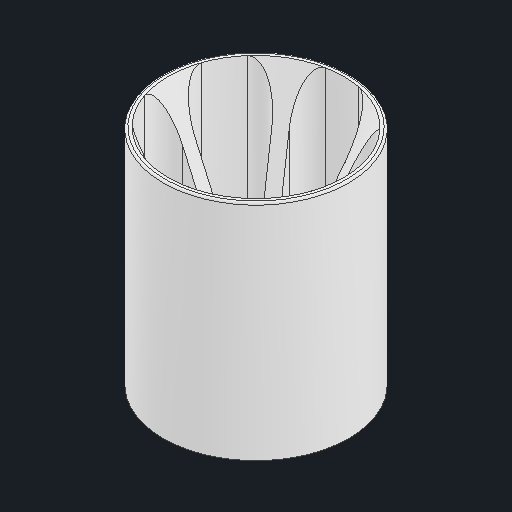
# Autodesk Inventor part: felga
Saved by Autodesk Inventor 2023 (Build 270158000, 158)
## iProperties
Created: 2024-06-08
Part Number: felga
Material: ABS Plastic
Document SubType Name: Modeling
Designer: szymo
Density: 1.06 g/cm^3
Appearance: Smooth - White
Mass: 25.2568 g
Surface Area: 203.005 cm^2
Volume: 23.8272 cm^3
Author: szymo
Autodesk Inventor part; units mm, degrees
ref_plane "YZ Plane" through (0, 0, 0) normal (1, 0, 0) x (0, 1, 0)
ref_plane "XZ Plane" through (0, 0, 0) normal (0, 1, 0) x (-1, 0, 0)
ref_plane "XY Plane" through (0, 0, 0) normal (0, 0, 1) x (1, 0, 0)
sketch "Sketch1" plane through (0, 0, 0) normal (0, 1, 0) x (-1, 0, 0)
  circle A0 centre (0, 0) radius 25
  circle A1 centre (0, 0) radius 22
  circle A2 centre (0, 0) radius 20.8
  dimension "d0" = 50
  dimension "d1" = 3
  dimension "d2" = 1.2
  constraints: 3 centre point, 3 coincident
  measures "d0" diameter of A0
  measures "d1" radial gap between concentric circles of A0 A1
  measures "d2" radial gap between concentric circles of A1 A2
extrude "Extrusion1" add sketch "Sketch1" along normal blind 53 contours A1
sketch "Sketch2" plane through (0, 0, 0) normal (0, 1, 0) x (-1, 0, 0)
  circle A0 centre (0, 0) radius 22 projected
  circle A1 centre (0, 0) radius 20.8 projected
  circle A2 centre (0, 0) radius 5
  line L0 (0, 0) -> (20.8, 0) construction
  circle A3 centre (0, 0) radius 20.8 projected
  line L1 (4.7697, 1.5) -> (20.7458, 1.5)
  line L2 (20.7458, -1.5) -> (4.7697, -1.5)
  line L3 (1.0858, 4.8807) -> (9.0739, 18.7164)
  line L4 (0, 0) -> (10.4, 18.0133) construction
  line L5 (11.672, 17.2164) -> (3.6839, 3.3807)
  line L6 (-3.6839, 3.3807) -> (-11.672, 17.2164)
  line L7 (0, 0) -> (-10.4, 18.0133) construction
  line L8 (-9.0739, 18.7164) -> (-1.0858, 4.8807)
  line L9 (-4.7697, -1.5) -> (-20.7458, -1.5)
  line L10 (0, 0) -> (-20.8, 0) construction
  line L11 (-20.7458, 1.5) -> (-4.7697, 1.5)
  line L12 (-1.0858, -4.8807) -> (-9.0739, -18.7164)
  line L13 (0, 0) -> (-10.4, -18.0133) construction
  line L14 (-11.672, -17.2164) -> (-3.6839, -3.3807)
  line L15 (3.6839, -3.3807) -> (11.672, -17.2164)
  line L16 (0, 0) -> (10.4, -18.0133) construction
  line L17 (9.0739, -18.7164) -> (1.0858, -4.8807)
  point P0 (3.6839, 3.3807)
  point P1 (11.672, 17.2164)
  point P2 (9.0739, 18.7164)
  point P3 (1.0858, 4.8807)
  point P4 (-1.0858, 4.8807)
  point P5 (-9.0739, 18.7164)
  point P6 (-11.672, 17.2164)
  point P7 (-3.6839, 3.3807)
  point P8 (-4.7697, 1.5)
  point P9 (-20.7458, 1.5)
  point P10 (-4.7697, -1.5)
  point P11 (-3.6839, -3.3807)
  point P12 (-9.0739, -18.7164)
  point P13 (-1.0858, -4.8807)
  point P14 (1.0858, -4.8807)
  point P15 (9.0739, -18.7164)
  point P16 (3.6839, -3.3807)
  dimension "d5" = 10
  dimension "d6" = 1.5
  dimension "d7" = 1.5
  dimension "d10" = 360
  constraints: 36 end point, 5 point on circle, 2 parallel, 1 centre point, 1 coincident, 1 horizontal, 55 other
  measures "d5" diameter of A2
  measures "d6" distance between parallel lines of L1 L0
  measures "d7" distance between parallel lines of L0 L2
extrude "Extrusion2" add sketch "Sketch2" along normal blind 17 contours A1 L2 A2 L1 | L5 A2 L3 A1 | A2 | A1 L17 A2 L15 | L8 A2 L6 A1 | A1 L14 A2 L12 | L11 A2 L9 A1
chamfer "Chamfer1" distance 36 distance2 15.8 7 edges at (10.4, 17, 18.0133) (20.8, 17, 0) (10.4, 17, -18.0133) (-10.4, 17, -18.0133) (-20.7865, 17, 0.7505) (-20.7865, 17, -0.7505) (-10.4, 17, 18.0133) measured on face at (10.4, 17.5, 18.0133) measured on face at (-10.4, 17.5, -18.0133) measured on face at (-20.7865, 17.5, -0.7505) measured on face at (-20.7865, 17.5, 0.7505) measured on face at (20.8, 17.5, 0) measured on face at (-10.4, 17.5, 18.0133) measured on face at (10.4, 17.5, -18.0133)
sketch "Sketch3" plane through (0, 0, 0) normal (0, -1, 0) x (1, 0, 0)
  circle A0 centre (0, 0) radius 3
  line L0 (-2.0396, 2.2) -> (2.0396, 2.2)
  line L1 (2.0396, -2.2) -> (-2.0396, -2.2)
  dimension "d19" = 6
  dimension "d20" = 4.4
  dimension "d21" = 2.2
  dimension "d22" = 2.2
  constraints: 4 end point, 4 point on circle, 1 centre point, 1 coincident, 1 horizontal, 1 parallel
  measures "d19" diameter of A0
  measures "d20" distance between parallel lines of L0 L1
  measures "d21" distance from line of L0 point (0, 0)
  measures "d22" distance from line of L1 point (0, 0)
extrude "Extrusion3" cut sketch "Sketch3" against normal blind 12 contours A0 L1 L0
sketch "Sketch6" plane through (0, 0, 0) normal (0, -1, 0) x (1, 0, 0)
  circle A0 centre (0, 0) radius 22 projected
  circle A1 centre (0, -10) radius 3.5
  arc A2 (-9.0739, -18.7164) -> (9.0739, -18.7164) centre (0, 0) ccw projected
  arc A3 (-9.0739, -18.7164) -> (9.0739, -18.7164) centre (0, 0) ccw projected
  circle A4 centre (0, -14.8667) radius 5.9333
  circle A5 centre (12.8749, -7.4333) radius 5.9333
  circle A6 centre (8.6603, -5) radius 3.5
  circle A7 centre (12.8749, 7.4333) radius 5.9333
  circle A8 centre (8.6603, 5) radius 3.5
  circle A9 centre (0, 14.8667) radius 5.9333
  circle A10 centre (0, 10) radius 3.5
  circle A11 centre (-12.8749, 7.4333) radius 5.9333
  circle A12 centre (-8.6603, 5) radius 3.5
  circle A13 centre (-12.8749, -7.4333) radius 5.9333
  circle A14 centre (-8.6603, -5) radius 3.5
  line L0 (-1.0858, -4.8807) -> (-9.0739, -18.7164) projected
  arc A15 (-1.0858, -4.8807) -> (1.0858, -4.8807) centre (0, 0) ccw projected
  line L1 (9.0739, -18.7164) -> (1.0858, -4.8807) projected
  arc A16 (-1.0858, 4.8807) -> (-3.6839, 3.3807) centre (0, 0) ccw projected
  arc A17 (1.0858, 4.8807) -> (-1.0858, 4.8807) centre (0, 0) ccw projected
  arc A18 (3.6839, 3.3807) -> (1.0858, 4.8807) centre (0, 0) ccw projected
  arc A19 (4.7697, 1.5) -> (3.6839, 3.3807) centre (0, 0) ccw projected
  arc A20 (4.7697, -1.5) -> (4.7697, 1.5) centre (0, 0) ccw projected
  arc A21 (3.6839, -3.3807) -> (4.7697, -1.5) centre (0, 0) ccw projected
  arc A22 (1.0858, -4.8807) -> (3.6839, -3.3807) centre (0, 0) ccw projected
  arc A23 (-1.0858, -4.8807) -> (1.0858, -4.8807) centre (0, 0) ccw projected
  arc A24 (-3.6839, -3.3807) -> (-1.0858, -4.8807) centre (0, 0) ccw projected
  arc A25 (-4.7697, -1.5) -> (-3.6839, -3.3807) centre (0, 0) ccw projected
  arc A26 (-4.7697, 1.5) -> (-4.7697, -1.5) centre (0, 0) ccw projected
  arc A27 (-3.6839, 3.3807) -> (-4.7697, 1.5) centre (0, 0) ccw projected
  line L2 (-2.0396, 2.2) -> (2.0396, 2.2) projected
  arc A28 (2.0396, -2.2) -> (2.0396, 2.2) centre (0, 0) ccw projected
  line L3 (2.0396, -2.2) -> (-2.0396, -2.2) projected
  arc A29 (-2.0396, 2.2) -> (-2.0396, -2.2) centre (0, 0) ccw projected
  arc A30 (-9.0739, -18.7164) -> (9.0739, -18.7164) centre (0, 0) ccw projected
  line L4 (-1.0858, -4.8807) -> (-9.0739, -18.7164) projected
  arc A31 (-1.0858, -4.8807) -> (1.0858, -4.8807) centre (0, 0) ccw projected
  line L5 (9.0739, -18.7164) -> (1.0858, -4.8807) projected
  line L6 (3.6839, -3.3807) -> (11.672, -17.2164) projected
  arc A32 (3.6839, -3.3807) -> (4.7697, -1.5) centre (0, 0) ccw projected
  line L7 (20.7458, -1.5) -> (4.7697, -1.5) projected
  arc A33 (11.672, -17.2164) -> (20.7458, -1.5) centre (0, 0) ccw projected
  line L8 (4.7697, 1.5) -> (20.7458, 1.5) projected
  arc A34 (4.7697, 1.5) -> (3.6839, 3.3807) centre (0, 0) ccw projected
  line L9 (11.672, 17.2164) -> (3.6839, 3.3807) projected
  arc A35 (20.7458, 1.5) -> (11.672, 17.2164) centre (0, 0) ccw projected
  line L10 (1.0858, 4.8807) -> (9.0739, 18.7164) projected
  arc A36 (1.0858, 4.8807) -> (-1.0858, 4.8807) centre (0, 0) ccw projected
  line L11 (-9.0739, 18.7164) -> (-1.0858, 4.8807) projected
  arc A37 (9.0739, 18.7164) -> (-9.0739, 18.7164) centre (0, 0) ccw projected
  line L12 (-3.6839, 3.3807) -> (-11.672, 17.2164) projected
  arc A38 (-3.6839, 3.3807) -> (-4.7697, 1.5) centre (0, 0) ccw projected
  line L13 (-20.7458, 1.5) -> (-4.7697, 1.5) projected
  arc A39 (-11.672, 17.2164) -> (-20.7458, 1.5) centre (0, 0) ccw projected
  circle A40 centre (0, 0) radius 22 projected
  line L14 (-4.7697, -1.5) -> (-20.7458, -1.5) projected
  arc A41 (-4.7697, -1.5) -> (-3.6839, -3.3807) centre (0, 0) ccw projected
  line L15 (-11.672, -17.2164) -> (-3.6839, -3.3807) projected
  arc A42 (-20.7458, -1.5) -> (-11.672, -17.2164) centre (0, 0) ccw projected
  point P0 (0, -20.8)
  point P1 (3.0311, -8.25)
  point P2 (-3.0311, -8.25)
  point P3 (8.6603, -1.5)
  point P4 (4.7697, -1.5)
  point P5 (3.6839, -3.3807)
  point P6 (5.6292, -6.75)
  point P7 (5.6292, 6.75)
  point P8 (3.6839, 3.3807)
  point P9 (8.6603, 1.5)
  point P10 (-3.0311, 8.25)
  point P11 (-1.0858, 4.8807)
  point P12 (1.0858, 4.8807)
  point P13 (3.0311, 8.25)
  point P14 (-8.6603, 1.5)
  point P15 (-4.7697, 1.5)
  point P16 (-3.6839, 3.3807)
  point P17 (-5.6292, 6.75)
  point P18 (-5.6292, -6.75)
  point P19 (-3.6839, -3.3807)
  point P20 (-4.7697, -1.5)
  point P21 (-8.6603, -1.5)
  dimension "d40" = 7
  dimension "d51" = 360
  constraints: 12 centre point, 1 tangent, 25 other
  measures "d40" diameter of A1
extrude "fillleeciki" add sketch "Sketch6" against normal up to surface contours A1 L0 A15 L1 | A21 L7 A6 L6 | L15 A14 L14 A25 | A19 L9 A8 L8 | L13 A12 L12 A27 | A17 L11 A10 L10 round surface about axis through (0, 35, 0) along (0, 1, 0) radius 12.9 half angle 23.696137 far side no
sketch "Sketch5" plane through (0, 17, 0) normal (0, 1, 0) x (1, 0, 0)
  point P0 (0, 0)
  point P1 (0, 0)
  constraints: 1 coincident
hole "Hole2" at (0, 17, 0) direction (0, -1, 0) diameter 3.6 end through all counterbore diameter 6.5 counterbore depth 0 clearance for "Slotted Cheese Head Screw ISO 1207" size "M3" standard "ISO"
fillet "Fillet3" radius 0.5 1 edges at (22, 53, 0)
fillet "Fillet4" radius 4 12 edges at (-9.0739, 26.4999, -18.7164) (9.0739, 26.4999, -18.7164) (11.672, 26.4999, -17.2164) (20.7458, 26.4999, -1.5) (20.7458, 26.4999, 1.5) (11.672, 26.4999, 17.2164) (9.0739, 26.4999, 18.7164) (-11.672, 26.4999, 17.2164) (-9.0739, 26.4999, 18.7164) (-20.7458, 26.4999, -1.5) (-20.7458, 26.4999, 1.5) (-11.672, 26.4999, -17.2164)
equation "\"d7\" = d6"
equation "\"d21\" = d22"
body "Solid1"
